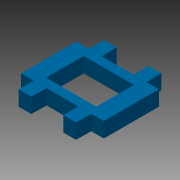
# Autodesk Inventor part: zCarNutHolder
Saved by Autodesk Inventor 2013 (Build 170138000, 138)
## iProperties
Created: 2015-01-14
Part Number: zCarNutHolder
Material: Generic
Document SubType Name: Modeling
Designer: dzban
Density: 1 g/cm^3
Author: dzban
Autodesk Inventor part; units mm, degrees
ref_plane "YZ Plane" through (0, 0, 0) normal (1, 0, 0) x (0, 1, 0)
ref_plane "XZ Plane" through (0, 0, 0) normal (0, 1, 0) x (-1, 0, 0)
ref_plane "XY Plane" through (0, 0, 0) normal (0, 0, 1) x (1, 0, 0)
sketch "Sketch1" plane through (0, 0, 0) normal (0, 0, 1) x (1, 0, 0)
  line L0 (19.6541, 4.0746) -> (19.6541, -10.9254)
  line L1 (19.6541, -10.9254) -> (-0.3459, -10.9254)
  line L2 (-0.3459, -10.9254) -> (-0.3459, 4.0746)
  line L3 (-0.3459, 4.0746) -> (19.6541, 4.0746)
  line L4 (-6.8459, 7.5746) -> (-6.8459, -14.4254)
  line L5 (-6.8459, -14.4254) -> (-1.8459, -14.4254)
  line L6 (-1.8459, -14.4254) -> (-1.7459, -20.4254)
  line L7 (-1.7459, -20.4254) -> (3.2541, -20.4254)
  line L8 (3.2541, -20.4254) -> (3.3541, -14.4254)
  line L9 (3.3541, -14.4254) -> (15.9541, -14.4254)
  line L10 (15.9541, -14.4254) -> (16.0541, -20.4254)
  line L11 (16.0541, -20.4254) -> (21.0541, -20.4254)
  line L12 (21.0541, -20.4254) -> (21.1541, -14.4254)
  line L13 (21.1541, -14.4254) -> (26.1541, -14.4254)
  line L14 (26.1541, -14.4254) -> (26.1541, 7.56)
  line L15 (26.1541, 7.56) -> (21.1536, 7.56)
  line L16 (21.1536, 7.56) -> (21.0538, 13.56)
  line L17 (21.0538, 13.56) -> (16.0538, 13.56)
  line L18 (16.0538, 13.56) -> (15.9541, 7.5746)
  line L19 (15.9541, 7.5746) -> (3.3541, 7.5746)
  line L20 (3.3541, 7.5746) -> (3.2541, 13.5746)
  line L21 (3.2541, 13.5746) -> (-1.7459, 13.5746)
  line L22 (-1.7459, 13.5746) -> (-1.8459, 7.5746)
  line L23 (-1.8459, 7.5746) -> (-6.8459, 7.5746)
  point P0 (0, 0)
  point P1 (0, 0)
  constraints: 48 end point
extrude "Extrusion1" add sketch "Sketch1" along normal blind 6
body "Solid1"
